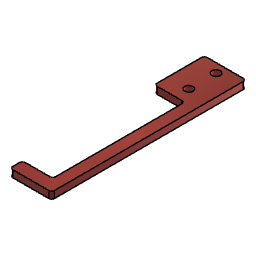
230414 replacement of broken part (Autodesk Fusion 360 design; units mm, degrees)
Autodesk Fusion 360 part; units mm, degrees
sketch "Sketch1" plane through (0, 0, 0) normal (0, 1, 0) x (1, 0, 0)
  line L0 (0, 0) -> (-30, 0)
  line L1 (-30, 0) -> (-30, -36)
  line L2 (0, -140) -> (0, 0)
  line L3 (0, -140) -> (-30, -140)
  line L4 (-30, -140) -> (-30, -131)
  line L5 (-30, -131) -> (-8.2, -131)
  line L6 (-8.2, -131) -> (-8.2, -36)
  line L7 (-30, -36) -> (-8.2, -36)
  circle A0 centre (-15, -26.14) radius 3
  circle A1 centre (-15, -6.54) radius 3
  dimension "d1" = 140
  dimension "d2" = 36
  dimension "d3" = 30
  dimension "d4" = 9
  dimension "d5" = 8.2
  dimension "d6" = 30
  dimension "d7" = 6
  dimension "d8" = 15
  dimension "d10" = 6
  dimension "d11" = 15
  dimension "d12" = 9.86
  dimension "d13" = 19.6
  constraint horizontal L0
  constraint vertical L1
  constraint vertical L2
  constraint coincident L0.start L2.end
  constraint perpendicular L2 L3
  constraint perpendicular L3 L4
  constraint perpendicular L4 L5
  constraint perpendicular L5 L6
  constraint perpendicular L1 L7
  measures "d1" distance of L0.start L2.start
  measures "d2" distance of L0.end L1.end
  measures "d3" distance of L2.start L3.end
  measures "d4" distance of L3.end L4.end
  measures "d5" distance of L2 L6
  measures "d6" distance of L0.start L0.end
  measures "d7" diameter of A0
  measures "d8" distance of L2 A0.centre
  measures "d10" diameter of A1
  measures "d11" distance of L2 A1.centre
  measures "d12" distance of L7 A0.centre
  measures "d13" distance of A0.centre A1.centre
extrude "Extrude1" add sketch "Sketch1" along normal blind 5
fillet "Fillet1" radius 2 8 edges at (-8.2, 2.5, 131) (-8.2, 2.5, 36) (-30, 2.5, 36) (-30, 2.5, 0) (0, 2.5, 0) (0, 2.5, 140) (-30, 2.5, 140) (-30, 2.5, 131)
